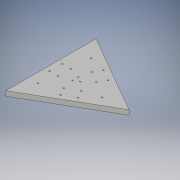
# Autodesk Inventor part: TraingleFifteen
Saved by Autodesk Inventor 2016 (Build 200138000, 138)
## iProperties
Created: 2017-04-26
Part Number: TraingleFifteen
Material: Generic
Document SubType Name: Modeling
Designer: Evan Phil George
Density: 1 g/cm^3
Appearance: Default
Author: Evan Phil George
Autodesk Inventor part; units mm, degrees
ref_plane "YZ Plane" through (0, 0, 0) normal (1, 0, 0) x (0, 1, 0)
ref_plane "XZ Plane" through (0, 0, 0) normal (0, 1, 0) x (-1, 0, 0)
ref_plane "XY Plane" through (0, 0, 0) normal (0, 0, 1) x (1, 0, 0)
sketch "Sketch1" plane through (0, 0, 0) normal (0, 1, 0) x (-1, 0, 0)
  line L0 (0, 0) -> (-90, 0)
  line L1 (-162.8128, 0) -> (81.4064, 141)
  line L2 (81.4064, 141) -> (81.4064, -141)
  line L3 (81.4064, -141) -> (-162.8128, 0)
  dimension "d0" = 90
  dimension "d1" = 282
  constraints: 8 end point, 1 coincident, 1 horizontal, 1 point on line, 7 other
  measures "d0" distance of L0.start L0.end
  measures "d1" distance of L2.end L1.start
extrude "TriangleFace" add sketch "Sketch1" along normal blind 15
sketch "Sketch2" plane through (0, 15, 0) normal (0, 1, 0) x (1, 0, 0)
  line L0 (-81.4064, 141) -> (-81.4064, -141) projected
  line L1 (-81.4064, 0) -> (-65.9064, 0)
  line L2 (-65.9064, 0) -> (-65.9064, 20)
  line L3 (-65.9064, 0) -> (-65.9064, -20)
  line L4 (-65.9064, 0) -> (-38.9064, 0)
  line L5 (-38.9064, 0) -> (-38.9064, 20)
  line L6 (-38.9064, 0) -> (-38.9064, -20)
  circle A0 centre (-65.9064, 20) radius 2
  circle A1 centre (-38.9064, 20) radius 2
  circle A2 centre (-65.9064, -20) radius 2
  circle A3 centre (-38.9064, -20) radius 2
  point P0 (0, 0)
  dimension "d4" = 15.5
  dimension "d5" = 20
  dimension "d6" = 20
  dimension "d7" = 27
  dimension "d8" = 20
  dimension "d9" = 20
  dimension "d10" = 4
  dimension "d11" = 4
  dimension "d12" = 4
  dimension "d13" = 4
  constraints: 12 end point, 4 centre point, 4 coincident, 3 vertical, 2 horizontal, 1 midpoint, 1 perpendicular
  measures "d4" distance of L1.start L1.end
  measures "d5" distance of L1.end L2.end
  measures "d6" distance of L1.end L3.end
  measures "d7" distance of L1.end L4.end
  measures "d8" distance of L4.end L5.end
  measures "d9" distance of L4.end L6.end
  measures "d10" diameter of A0
  measures "d11" diameter of A1
  measures "d12" diameter of A2
  measures "d13" diameter of A3
extrude "SideTwoHoles" cut sketch "Sketch2" against normal blind 15
sketch "Sketch3" plane through (0, 15, 0) normal (0, 1, 0) x (1, 0, 0)
  line L0 (162.8128, 0) -> (-81.4064, 141) projected
  line L1 (40.7032, 70.5) -> (32.9532, 57.0766)
  line L2 (32.9532, 57.0766) -> (19.4532, 33.6939)
  line L3 (32.9532, 57.0766) -> (15.6327, 67.0766)
  line L4 (32.9532, 57.0766) -> (50.2737, 47.0766)
  line L5 (19.4532, 33.6939) -> (2.1327, 43.6939)
  line L6 (19.4532, 33.6939) -> (36.7737, 23.6939)
  circle A0 centre (15.6327, 67.0766) radius 2
  circle A1 centre (50.2737, 47.0766) radius 2
  circle A2 centre (2.1327, 43.6939) radius 2
  circle A3 centre (36.7737, 23.6939) radius 2
  point P0 (0, 0)
  dimension "d16" = 15.5
  dimension "d17" = 27
  dimension "d18" = 20
  dimension "d19" = 20
  dimension "d20" = 20
  dimension "d21" = 20
  dimension "d22" = 4
  dimension "d23" = 4
  dimension "d24" = 4
  dimension "d25" = 4
  constraints: 12 end point, 5 perpendicular, 4 centre point, 4 coincident, 1 collinear, 1 midpoint
  measures "d16" distance of L1.start L1.end
  measures "d17" distance of L1.end L2.end
  measures "d18" distance of L1.end L3.end
  measures "d19" distance of L1.end L4.end
  measures "d20" distance of L2.end L5.end
  measures "d21" distance of L2.end L6.end
  measures "d22" diameter of A0
  measures "d23" diameter of A1
  measures "d24" diameter of A2
  measures "d25" diameter of A3
extrude "SideOneHoles" cut sketch "Sketch3" against normal blind 15
sketch "Sketch4" plane through (0, 15, 0) normal (0, 1, 0) x (1, 0, 0)
  line L0 (-81.4064, -141) -> (162.8128, 0) projected
  line L1 (40.7032, -70.5) -> (32.9532, -57.0766)
  line L2 (32.9532, -57.0766) -> (19.4532, -33.6939)
  line L3 (19.4532, -33.6939) -> (36.7737, -23.6939)
  line L4 (19.4532, -33.6939) -> (2.1327, -43.6939)
  line L5 (32.9532, -57.0766) -> (50.2737, -47.0766)
  line L6 (32.9532, -57.0766) -> (15.6327, -67.0766)
  circle A0 centre (36.7737, -23.6939) radius 2
  circle A1 centre (2.1327, -43.6939) radius 2
  circle A2 centre (50.2737, -47.0766) radius 2
  circle A3 centre (15.6327, -67.0766) radius 2
  point P0 (0, 0)
  dimension "d28" = 15.5
  dimension "d29" = 27
  dimension "d30" = 20
  dimension "d31" = 20
  dimension "d32" = 20
  dimension "d33" = 20
  dimension "d34" = 4
  dimension "d35" = 4
  dimension "d36" = 4
  dimension "d37" = 4
  constraints: 12 end point, 4 centre point, 4 coincident, 4 perpendicular, 1 collinear, 1 midpoint, 1 point on line
  measures "d28" distance of L1.start L1.end
  measures "d29" distance of L1.end L2.end
  measures "d30" distance of L2.end L3.end
  measures "d31" distance of L2.end L4.end
  measures "d32" distance of L1.end L5.end
  measures "d33" distance of L1.end L6.end
  measures "d34" diameter of A0
  measures "d35" diameter of A1
  measures "d36" diameter of A2
  measures "d37" diameter of A3
extrude "SideThreeHoles" cut sketch "Sketch4" against normal blind 15
sketch "Sketch5" plane through (0, 15, 0) normal (0, 1, 0) x (1, 0, 0)
  line L0 (-81.4064, -141) -> (162.8128, 0) projected
  line L1 (162.8128, 0) -> (-81.4064, 141) projected
  line L2 (162.8128, 0) -> (-81.4064, 0)
  line L3 (-81.4064, 141) -> (-81.4064, -141) projected
  line L4 (17.3205, 0) -> (-8.6603, -15)
  line L5 (-8.6603, -15) -> (-8.6603, 15)
  line L6 (-8.6603, 15) -> (17.3205, 0)
  line L7 (-8.6603, 15) -> (-5.1603, 8.9378)
  line L8 (-8.6603, 15) -> (-1.6603, 15) construction
  circle A0 centre (-5.1603, 8.9378) radius 1.75
  line L9 (-8.6603, -15) -> (-5.1603, -8.9378)
  line L10 (-8.6603, -15) -> (-1.6603, -15) construction
  circle A1 centre (-5.1603, -8.9378) radius 1.75
  line L11 (17.3205, 0) -> (10.3205, 0)
  line L12 (17.3205, 0) -> (24.3205, 0) construction
  circle A2 centre (10.3205, 0) radius 1.75
  point P0 (0, 0)
  point P1 (0, 0)
  dimension "d40" = 30
  dimension "d43" = 7
  dimension "d44" = 60
  dimension "d45" = 3.5
  dimension "d46" = 7
  dimension "d47" = 60
  dimension "d48" = 3.5
  dimension "d49" = 7
  dimension "d50" = 180
  dimension "d51" = 3.5
  constraints: 20 end point, 4 coincident, 3 centre point, 3 equal length, 3 horizontal, 1 collinear, 1 midpoint, 1 point on line, 7 other
  measures "d40" distance of L5.end L4.start
  measures "d43" distance of L5.end L7.end
  measures "d44" angle of L7 L8
  measures "d45" diameter of A0
  measures "d46" distance of L4.end L9.end
  measures "d47" angle of L10 L9
  measures "d48" diameter of A1
  measures "d49" distance of L4.start L11.end
  measures "d50" angle of L11 L12
  measures "d51" diameter of A2
extrude "CenterHoles" cut sketch "Sketch5" against normal blind 15 contours A1 | A0 | A2 L2 | L2 A2
sketch "Sketch6" plane through (0, 15, 0) normal (0, 1, 0) x (1, 0, 0)
  line L0 (-81.4064, -141) -> (162.8128, 0) projected
  line L1 (-81.4064, -141) -> (-81.4064, -71)
  line L2 (-81.4064, 141) -> (-81.4064, -141) projected
  line L3 (-81.4064, -71) -> (-51.4064, -71)
  line L4 (-81.4064, -71) -> (-51.4064, -71) construction
  circle A0 centre (-51.4064, -71) radius 2
  line L5 (162.8128, 0) -> (-81.4064, 141) projected
  line L6 (-81.4064, 141) -> (-20.7846, 106)
  line L7 (-20.7846, 106) -> (-35.7846, 80.0192)
  line L8 (162.8128, 0) -> (102.191, -35)
  line L9 (102.191, -35) -> (87.191, -9.0192)
  circle A1 centre (-35.7846, 80.0192) radius 2
  circle A2 centre (87.191, -9.0192) radius 2
  point P0 (0, 0)
  dimension "d54" = 70
  dimension "d55" = 30
  dimension "d56" = 0
  dimension "d57" = 4
  dimension "d60" = 70
  dimension "d61" = 30
  dimension "d62" = 70
  dimension "d63" = 30
  dimension "d64" = 4
  dimension "d65" = 4
  constraints: 14 end point, 3 centre point, 3 coincident, 3 point on line, 2 horizontal, 2 perpendicular, 1 collinear
  measures "d54" distance of L0.start L1.end
  measures "d55" distance of L1.end L3.end
  measures "d56" distance between parallel lines of L3 L4
  measures "d57" diameter of A0
  measures "d60" distance of L2.start L6.end
  measures "d61" distance of L6.end L7.end
  measures "d62" distance of L0.end L8.end
  measures "d63" distance of L8.end L9.end
  measures "d64" diameter of A1
  measures "d65" diameter of A2
extrude "Extrusion7" cut sketch "Sketch6" against normal blind 15 contours A2 | A1 | A0
body "Solid1"
